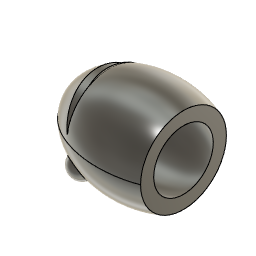
turtle_head v5 (Autodesk Fusion 360 design; units mm, degrees)
Autodesk Fusion 360 part; units mm, degrees
note: some values were not read from the file. Set by a fixed rule: which sketch regions a step uses.
sketch "Sketch5" plane through (0, 0, 0) normal (0, 0, 1) x (1, 0, 0)
  ellipse E0 centre (0, 0) end of major axis (-30, 0) minor radius 20
  line L0 (30, 0) -> (-30, 0)
  line L1 (0, 20) -> (0, -20)
  ellipse E1 centre (0, 0) end of major axis (-25, 0) minor radius 15
  line L2 (25, 0) -> (-25, 0)
  line L3 (0, 15) -> (0, -15)
  line L4 (14.9075, -17.356) -> (14.9075, 17.356)
  line L5 (-30, 0) -> (-25, 0)
  dimension "d13" = 30
  dimension "d14" = 20
  dimension "d15" = 5
  dimension "d16" = 5
  constraint coincident E0.centre E1.centre
  constraint horizontal L0
  constraint coincident E0 L0.start
  constraint coincident E0 L0.end
  constraint coincident E0 L1.start
  constraint coincident E0 L1.end
  constraint concentric E0 E1
  constraint perpendicular L1 L2
  constraint coincident E1 L2.start
  constraint coincident E1 L2.end
  constraint coincident E1 L3.start
  constraint coincident E1 L3.end
  constraint coincident E0 L4.start
  constraint coincident E0 L4.end
  constraint perpendicular L2 L4
  measures "d13" distance of E0.centre L0.end
  measures "d14" distance of E0.centre L1.start
  measures "d15" distance of L1.start L3.start
  measures "d16" distance of L0.end L2.end
revolve "Revolve6" add sketch "Sketch5" angle 360 about axis through (30, 0, 0) along (-1, 0, 0) contours E0 L0 L1 E1 L5 | E0 L1 E1 L4 picked at (-9.1963, -17.294) picked at (8.6022, -15.7103) makes body 1
sphere "SpherePrimitive2" add diameter 10 placed x (1, 0, 0) y (0, 1, 0) z (0, 0, 1) at (-8, 8, 0) separate body makes body 2
move_body "Move1" bodies 2 to x (1, 0, 0) y (0, 1, 0) z (0, 0, 1) at (-6, -20, -10)
mirror "Mirror1" about plane through (0, 0, 0) normal (0, 1, 0) of bodies 2 makes body 3
ref_plane "WorkPlane1" through (-35, 0, 0) normal (1, 0, 0) x (0, 1, 0)
sketch "Sketch7" plane through (-35, 0, 0) normal (1, 0, 0) x (0, 1, 0)
  arc A0 (19.5297, 1.3117) -> (-19.5297, 1.3116) centre (0, -3) ccw
  arc A1 (17.5767, 0.8805) -> (19.5297, 1.3117) centre (18.5532, 1.0961) ccw
  arc A2 (17.5767, 0.8805) -> (-17.5767, 0.8805) centre (0, -3) ccw
  arc A3 (-19.5297, 1.3116) -> (-17.5767, 0.8805) centre (-18.5532, 1.0961) ccw
  arc A4 (18.5532, 1.0961) -> (-18.5532, 1.0961) centre (0, -3) ccw construction
  dimension "d25" = 20
  dimension "d26" = 2
  dimension "d27" = 37.1065
  constraint tangent A0 A1
  constraint tangent A1 A2
  constraint tangent A2 A3
  constraint tangent A0 A3
  measures "d25" radius of A0
  measures "d26" distance of A0 A2
  measures "d27" horizontal distance of A3.centre A1.centre
extrude "Extrude1" cut sketch "Sketch7" along normal blind 20 bodies 1
split "Split1" by bodies 1 bodies 2 3 makes body 6 at (-18.9761, 12.4557, -10.1743) makes body 7 at (-9.786, 9.3716, -9.4225) makes body 4 at (-18.9774, -12.426, -10.2098) makes body 5 at (-15.3629, -7.4413, -8.4635)
combine "Combine1" operation add target body 4 tool bodies 6 3 2 1
scale "Scale1" factor 1.35 about (-25, 0, 0) bodies 4
